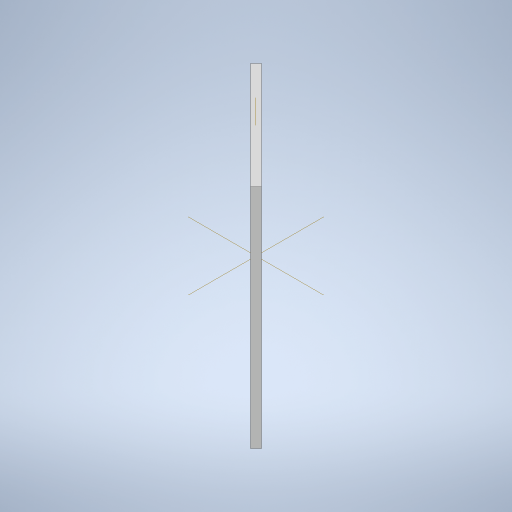
# Autodesk Inventor part: InclinePlate
Saved by Autodesk Inventor 2023.2 (Build 272271030, 271C)
## iProperties
Created: 2023-03-03
Part Number: InclinePlate
Material: Generisch
Document SubType Name: Modeling
Designer: mehan
Density: 1 g/cm^3
Appearance: Vorgabe
Author: mehan
Autodesk Inventor part; units mm, degrees
ref_plane "YZ Plane" through (0, 0, 0) normal (1, 0, 0) x (0, 1, 0)
ref_plane "XZ Plane" through (0, 0, 0) normal (0, 1, 0) x (-1, 0, 0)
ref_plane "XY Plane" through (0, 0, 0) normal (0, 0, 1) x (1, 0, 0)
sketch "Skizze1" plane through (0, 0, 0) normal (0, 1, 0) x (-1, 0, 0)
  line L0 (33.5876, -37.1231) -> (37.1231, -33.5876)
  line L1 (37.1231, -33.5876) -> (-33.5876, 37.1231)
  line L2 (-33.5876, 37.1231) -> (-37.1231, 33.5876)
  line L3 (-37.1231, 33.5876) -> (33.5876, -37.1231)
  line L4 (33.5876, -37.1231) -> (-33.5876, 37.1231) construction
  line L5 (37.1231, -33.5876) -> (-37.1231, 33.5876) construction
  line L6 (33.5876, -37.1231) -> (38.5876, -37.1231) construction
  point P0 (0, 0)
  dimension "d0" = 5
  dimension "d1" = 45
  dimension "d2" = 100
  constraints: 14 end point, 2 midpoint, 2 parallel, 1 equal length, 1 horizontal, 1 perpendicular
  measures "d0" distance of L0.start L0.end
  measures "d1" angle of L6 L0
  measures "d2" distance of L1.end L0.end
extrude "Extrusion1" add sketch "Skizze1" along normal mid plane 150
